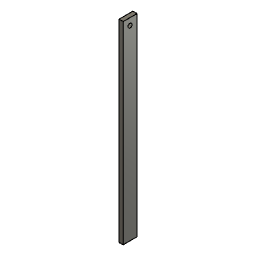
stamp support v1 (Autodesk Fusion 360 design; units mm, degrees)
Autodesk Fusion 360 part; units mm, degrees
sketch "Sketch1" plane through (0, 0, 0) normal (1, 0, 0) x (0, 0, -1)
  line L0 (-10, 140) -> (10, 140)
  line L1 (10, 140) -> (10, -140)
  line L2 (10, -140) -> (-10, -140)
  line L3 (-10, -140) -> (-10, 140)
  circle A0 centre (0, 130) radius 3
  dimension "d1" = 20
  dimension "d2" = 280
  dimension "d3" = 6
  dimension "d4" = 10
  constraint horizontal L0
  constraint perpendicular L0 L1
  constraint parallel L0 L2
  constraint parallel L1 L3
  measures "d1" distance of L1.end L2.end
  measures "d2" distance of L0.end L1.end
  measures "d3" diameter of A0
  measures "d4" distance of L0 A0.centre
extrude "Extrude1" add sketch "Sketch1" along normal blind 6
